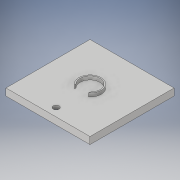
# Autodesk Inventor part: Tapapotenciometro_v1
Saved by Autodesk Inventor 2019 (Build 230136000, 136)
## iProperties
Created: 2020-06-11
Part Number: Tapapotenciometro_v1
Material: Genérico
Document SubType Name: Modeling
Designer: Samuel
Density: 1 g/cm^3
Appearance: Valor por defecto
Author: Samuel
Autodesk Inventor part; units mm, degrees
ref_plane "YZ Plane" through (0, 0, 0) normal (1, 0, 0) x (0, 1, 0)
ref_plane "XZ Plane" through (0, 0, 0) normal (0, 1, 0) x (-1, 0, 0)
ref_plane "XY Plane" through (0, 0, 0) normal (0, 0, 1) x (1, 0, 0)
sketch "Boceto1" plane through (0, 0, 0) normal (0, 1, 0) x (-1, 0, 0)
  line L0 (-36, 36) -> (36, 36)
  line L1 (36, 36) -> (36, -36)
  line L2 (36, -36) -> (-36, -36)
  line L3 (-36, -36) -> (-36, 36)
  line L4 (-36, 36) -> (36, -36) construction
  line L5 (36, 36) -> (-36, -36) construction
  line L6 (-34.5, 34.5) -> (34.5, 34.5)
  line L7 (34.5, 34.5) -> (34.5, -34.5)
  line L8 (34.5, -34.5) -> (-34.5, -34.5)
  line L9 (-34.5, -34.5) -> (-34.5, 34.5)
  line L10 (-34.5, 34.5) -> (34.5, -34.5) construction
  line L11 (34.5, 34.5) -> (-34.5, -34.5) construction
  point P0 (0, 0)
  dimension "d0" = 72
  dimension "d1" = 72
  dimension "d2" = 69
  dimension "d3" = 69
  constraints: 24 end point, 4 midpoint, 4 parallel, 2 horizontal, 2 perpendicular
  measures "d0" distance of L1.end L2.end
  measures "d1" distance of L0.end L1.end
  measures "d2" distance of L7.end L8.end
  measures "d3" distance of L6.end L7.end
extrude "Extrusión1" add sketch "Boceto1" along normal blind 3
sketch "Boceto2" plane through (0, 3, 0) normal (0, 1, 0) x (1, 0, 0)
  line L0 (-36, 36) -> (-36, -36) projected
  line L1 (-36, -36) -> (36, -36) projected
  line L2 (36, 36) -> (-36, 36) projected
  line L3 (36, -36) -> (36, 36) projected
  line L4 (36, -36) -> (-36, -36)
  line L5 (-36, -36) -> (-36, 36)
  line L6 (-36, 36) -> (36, 36)
  line L7 (36, 36) -> (36, -36)
  line L8 (36, -36) -> (-36, 36) construction
  line L9 (-36, -36) -> (36, 36) construction
  point P0 (0, 0)
  constraints: 12 end point, 2 midpoint, 2 parallel, 1 horizontal, 1 perpendicular
extrude "Extrusión2" add sketch "Boceto2" along normal blind 3
sketch "Boceto3" plane through (0, 6, 0) normal (0, 1, 0) x (1, 0, 0)
  line L0 (-36, 36) -> (-36, -36) projected
  line L1 (-36, -36) -> (36, -36) projected
  line L2 (36, -36) -> (36, 36) projected
  line L3 (36, 36) -> (-36, 36) projected
  circle A0 centre (0, -29) radius 2.5
  circle A1 centre (0, 0) radius 8.5
  circle A2 centre (0, 0) radius 9.5
  line L4 (6, -13) -> (-6, -5) construction
  line L5 (-6, -13) -> (6, -5) construction
  line L6 (-6, -7.3655) -> (-6, -6.0208)
  line L7 (6, -7.3655) -> (6, -6.0208)
  arc A3 (-6, -6.0208) -> (6, -6.0208) centre (0, 0) ccw
  arc A4 (-6, -7.3655) -> (6, -7.3655) centre (0, 0) ccw
  point P0 (0, -9)
  dimension "d8" = 5
  dimension "d9" = 17
  dimension "d10" = 19
  constraints: 8 end point, 8 point on circle, 5 centre point, 2 coincident, 2 concentric, 2 midpoint
  measures "d8" diameter of A0
  measures "d9" diameter of A1
  measures "d10" diameter of A2
extrude "Extrusión3" add sketch "Boceto3" along normal blind 3 contours A1 L6 A2 L7 picked at (9.0782, 0.7435)
sketch "Boceto4" plane through (0, 6, 0) normal (0, 1, 0) x (1, 0, 0)
  circle A0 centre (0, -29) radius 2.5
  point P0 (0, 0)
  dimension "d13" = 5
  constraints: 1 centre point
  measures "d13" diameter of A0
extrude "Extrusión4" cut sketch "Boceto4" against normal blind 3
